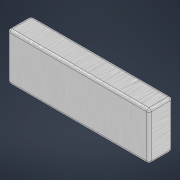
# Autodesk Inventor part: NS
Saved by Autodesk Inventor 2022 (Build 260153070, 153G)
## iProperties
Created: 2022-02-01
Part Number: NS
Material: Типовые
Document SubType Name: Modeling
Designer: kalugin_a
Density: 1 g/cm^3
Appearance: По умолчанию
Author: kalugin_a
Autodesk Inventor part; units mm, degrees
ref_plane "YZ Plane" through (0, 0, 0) normal (1, 0, 0) x (0, 1, 0)
ref_plane "XZ Plane" through (0, 0, 0) normal (0, 1, 0) x (-1, 0, 0)
ref_plane "XY Plane" through (0, 0, 0) normal (0, 0, 1) x (1, 0, 0)
sketch "Эскиз1" plane through (0, 0, 0) normal (0, 0, 1) x (1, 0, 0)
  line L0 (1, 0) -> (59, 0)
  line L1 (60, 1) -> (60, 19)
  line L2 (59, 20) -> (1, 20)
  line L3 (0, 19) -> (0, 1)
  arc A0 (1, 20) -> (0, 19) centre (1, 19) ccw
  arc A1 (59, 0) -> (60, 1) centre (59, 1) ccw
  arc A2 (60, 19) -> (59, 20) centre (59, 19) ccw
  arc A3 (0, 1) -> (1, 0) centre (1, 1) ccw
  point P0 (0, 0)
  point P1 (60, 20)
  point P2 (60, 0)
  point P3 (0, 20)
  dimension "d0" = 60
  dimension "d1" = 20
  dimension "d2" = 1
  dimension "d3" = 1
  constraints: 8 end point, 8 point on circle, 8 point on line, 8 tangent, 4 centre point, 2 equal radius, 2 parallel, 1 horizontal, 1 perpendicular
  measures "d0" distance of point (0, 20) point (60, 20)
  measures "d1" distance of point (60, 20) point (60, 0)
  measures "d2" radius of A0
  measures "d3" radius of A3
extrude "Выдавливание1" add sketch "Эскиз1" along normal blind 10
fillet "Сопряжение1" radius 1 16 edges at (0.2929, 19.7071, 10) (0, 10, 10) (0.2929, 0.2929, 10) (30, 0, 10) (59.7071, 0.2929, 10) (60, 10, 10) (59.7071, 19.7071, 10) (30, 20, 10) (59.7071, 19.7071, 0) (30, 20, 0) (0.2929, 19.7071, 0) (0, 10, 0) (0.2929, 0.2929, 0) (30, 0, 0) (59.7071, 0.2929, 0) (60, 10, 0)
